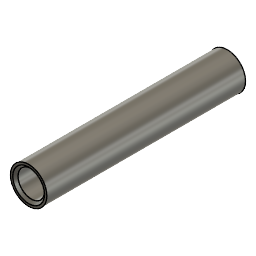
ESPAÇADOR_MID_TOP (Autodesk Fusion 360 design; units mm, degrees)
Autodesk Fusion 360 part; units mm, degrees
sketch "Esboço1" plane through (0, 0, 0) normal (0, 0, 1) x (1, 0, 0)
  circle A0 centre (0, 0) radius 3
  dimension "d1" = 6
  constraint coincident A0.centre origin
  measures "d1" diameter of A0
extrude "Extrusão1" add sketch "Esboço1" along normal blind 40
sketch "Esboço2" plane through (0, 0, 40) normal (0, 0, 1) x (1, 0, 0)
  circle A0 centre (0, 0) radius 3
  circle A1 centre (0, 0) radius 2
  dimension "d4" = 4
  constraint coincident A0.centre A1.centre
  measures "d4" diameter of A1
extrude "Extrusão2" cut sketch "Esboço2" against normal blind 4 contours A1
extrude "Extrusão3" cut 1 faces at (-1.1591, 0.5829, 0) along direction (0, 0, 1) blind 10
extrude "Extrusão4" cut 1 faces at (0.637, 0.1965, 36) along direction (0, 0, -1) blind 1
chamfer "Chanfro1" distance 0.4 angle 45 1 edges at (-1.8647, 0.7232, 40)
sketch "Esboço3" plane through (0, 0, 10) normal (0, 0, -1) x (-1, 0, 0)
  circle A0 centre (0, 0) radius 3
  circle A1 centre (0, 0) radius 1.4
  dimension "d12" = 2.8
  constraint coincident A0.centre A1.centre
  measures "d12" diameter of A1
extrude "Extrusão5" cut sketch "Esboço3" against normal blind 10 contours A1
sketch "Esboço4" plane through (0, 0, 10) normal (0, 0, -1) x (-1, 0, 0)
  circle A0 centre (0, 0) radius 1.4
  circle A1 centre (0, 0) radius 3
  circle A2 centre (0, 0) radius 3
  circle A3 centre (0, 0) radius 2.75
  dimension "d15" = 5.5
  constraint coincident A0.centre A1.centre
  measures "d15" diameter of A3
extrude "Extrusão6" cut sketch "Esboço4" against normal blind 34 contours A1 A2
extrude "Extrusão7" cut 1 faces at (0.637, 0.1965, 35) along direction (0, 0, -1) blind 1
